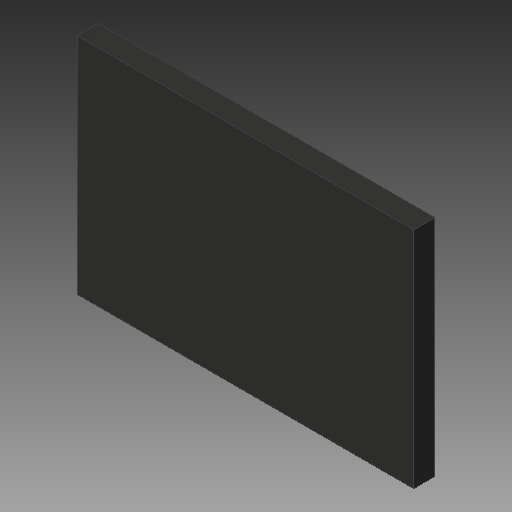
# Autodesk Inventor part: speaker-base-sorbothane
Saved by Autodesk Inventor 2019 (Build 230136000, 136)
## iProperties
Created: 2019-04-15
Part Number: speaker-base-sorbothane
Material: Rubber
Document SubType Name: Modeling
Designer: Wilson Lab
Density: 0.93 g/cm^3
Appearance: Rubber - Black
Author: Wilson Lab
Autodesk Inventor part; units mm, degrees
ref_plane "YZ Plane" through (0, 0, 0) normal (1, 0, 0) x (0, 1, 0)
ref_plane "XZ Plane" through (0, 0, 0) normal (0, 1, 0) x (-1, 0, 0)
ref_plane "XY Plane" through (0, 0, 0) normal (0, 0, 1) x (1, 0, 0)
ref_plane "Work Plane1" through (0, 0, 0) normal (0, 0, 1) x (1, 0, 0)
sketch "Sketch1" plane through (0, 0, 0) normal (0, 0, 1) x (1, 0, 0)
  line L0 (-63.5, -38.1) -> (-63.5, 38.1) construction
  line L1 (-19.05, -38.1) -> (-63.5, -38.1) construction
  line L2 (19.05, -38.1) -> (-19.05, -38.1) construction
  line L3 (63.5, -38.1) -> (19.05, -38.1) construction
  line L4 (63.5, 38.1) -> (63.5, -38.1) construction
  line L5 (19.05, 38.1) -> (63.5, 38.1) construction
  line L6 (-19.05, 38.1) -> (19.05, 38.1) construction
  line L7 (-63.5, 38.1) -> (-19.05, 38.1) construction
  line L8 (-76, 50.6) -> (-76, -50.6)
  line L9 (-76, -50.6) -> (-19.05, -50.6)
  line L10 (-19.05, -50.6) -> (19.05, -50.6)
  line L11 (19.05, -50.6) -> (76, -50.6)
  line L12 (76, -50.6) -> (76, 50.6)
  line L13 (76, 50.6) -> (19.05, 50.6)
  line L14 (19.05, 50.6) -> (-19.05, 50.6)
  line L15 (-19.05, 50.6) -> (-76, 50.6)
  point P0 (0, 0)
  dimension "d0" = 12.5
  constraints: 16 end point, 7 other
  measures "d0" distance between parallel lines of L14 L6
extrude "Extrusion1" add sketch "Sketch1" along normal blind 9.525
body "Solid1"
